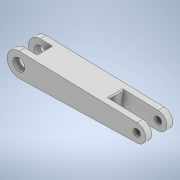
# Autodesk Inventor part: New_ThinArm_second
Saved by Autodesk Inventor 2021 (Build 250183000, 183)
## iProperties
Created: 2021-08-05
Part Number: New_ThinArm_second
Material: Generic
Document SubType Name: Modeling
Designer: hp
Density: 1 g/cm^3
Appearance: Default
Author: hp
Autodesk Inventor part; units mm, degrees
ref_plane "YZ Plane" through (0, 0, 0) normal (1, 0, 0) x (0, 1, 0)
ref_plane "XZ Plane" through (0, 0, 0) normal (0, 1, 0) x (-1, 0, 0)
ref_plane "XY Plane" through (0, 0, 0) normal (0, 0, 1) x (1, 0, 0)
sketch "Sketch1" plane through (0, 0, 0) normal (0, 0, 1) x (1, 0, 0)
  circle A0 centre (0, 0) radius 2
  circle A1 centre (0, 0) radius 1
  line L0 (0, 0) -> (20, 0)
  circle A2 centre (20, 0) radius 1.5
  circle A3 centre (20, 0) radius 0.6
  line L1 (0.05, 1.9994) -> (20.0375, 1.4995)
  line L2 (0.05, -1.9994) -> (20.0375, -1.4995)
  dimension "d0" = 4
  dimension "d1" = 2
  dimension "d2" = 20
  dimension "d3" = 3
  dimension "d4" = 1.2
  constraints: 6 end point, 4 centre point, 4 coincident, 4 point on circle, 4 tangent, 1 horizontal
  measures "d0" diameter of A0
  measures "d1" diameter of A1
  measures "d2" distance of L0.start L0.end
  measures "d3" diameter of A2
  measures "d4" diameter of A3
extrude "Extrusion1" add sketch "Sketch1" along normal mid plane 4.6
sketch "Sketch2" plane through (0, 0, 0) normal (0, 0, 1) x (1, 0, 0)
  line L0 (0, 0) -> (2, 0)
  line L1 (2, 0) -> (2, 1.9506)
  line L2 (20.0375, 1.4995) -> (0.05, 1.9994) projected
  line L3 (2, 0) -> (2, -1.9506)
  line L4 (0.05, -1.9994) -> (20.0375, -1.4995) projected
  circle A0 centre (0, 0) radius 2.5
  circle A1 centre (20, 0) radius 0.6 projected
  circle A2 centre (20, 0) radius 6
  point P0 (2, -1.5)
  point P1 (2, 1.5)
  point P2 (1.5495, 1.9619)
  point P3 (1.5495, -1.9619)
  dimension "d7" = 2
  dimension "d8" = 5
  dimension "d10" = 12
  constraints: 6 end point, 3 point on line, 2 centre point, 2 coincident, 1 horizontal, 1 vertical
  measures "d7" distance of L0.start L0.end
  measures "d8" diameter of A0
  measures "d10" diameter of A2
extrude "Extrusion2" cut sketch "Sketch2" along normal mid plane 2.6 contours L3 A0 L1 | L1 A0 L3 | A0 L2 L1 | L3 L4 A0 | A2
fillet "Fillet1" radius 0.1 4 edges at (2, 1.5, 0) (2, -1.5, 0) (2, 1.9506, 0) (2, -1.9506, 0)
fillet "Fillet2" radius 0.2 2 edges at (14.2298, 1.6448, 0) (14.2298, -1.6448, 0)
body "Solid1"
